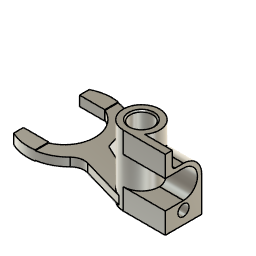
22 (Autodesk Fusion 360 design; units mm, degrees)
Autodesk Fusion 360 part; units mm, degrees
note: some values were not read from the file. Chosen so that the rebuilt part matches the saved one: where a step ends.
sketch "草图1" plane through (0, 0, 0) normal (0, 0, 1) x (1, 0, 0)
  line L0 (-13.1652, 20) -> (4.8348, 20)
  line L1 (-13.1652, -20) -> (4.8348, -20)
  line L2 (-40, 0) -> (55, 0) construction
  line L3 (-13.1652, 20) -> (-13.1652, 26.957)
  line L4 (-13.1652, -20) -> (-13.1652, -26.957)
  line L5 (-13.1652, -20) -> (4.8348, -20)
  line L6 (4.8348, -20) -> (4.8348, -29.6078)
  line L7 (4.8348, 20) -> (4.8348, 29.6078)
  arc A0 (-13.1652, -26.957) -> (-13.1652, 26.957) centre (0, 0) ccw
  arc A1 (4.8348, -20.1481) -> (4.8348, 20.1481) centre (-4, 0) ccw
  line L8 (13.7832, 26.6462) -> (71.9727, -3.4533)
  line L9 (62.4167, -27.4964) -> (31.174, -18.5377)
  arc A2 (31.174, -18.5377) -> (21.3132, -21.1127) centre (28.4176, -28.1503) ccw
  circle A3 centre (66, -15) radius 13
  circle A4 centre (66, -15) radius 8
  point P0 (66, -15)
  dimension "d5" = 60
  dimension "d6" = 44
  dimension "d7" = 4
  dimension "d8" = 20
  dimension "d9" = 40
  dimension "d10" = 18
  dimension "d11" = 18
  dimension "d13" = 15
  dimension "d14" = 10
  dimension "d16" = 70
  dimension "d17" = 26
  dimension "d18" = 16
  dimension "d19" = 16
  constraint coincident A0.centre origin
  constraint horizontal L0
  constraint parallel L0 L1
  constraint horizontal L2
  constraint collinear A1.centre L2.start L2.end
  constraint perpendicular L0 L3
  constraint perpendicular L1 L4
  constraint coincident L6.end A0
  constraint perpendicular L1 L6
  constraint coincident L7.end A0
  constraint perpendicular L0 L7
  constraint coincident L7 A1.end
  constraint coincident L6 A1.start
  constraint coincident A0 L8.start
  constraint coincident A0 A2.end
  constraint tangent L9 A2
  constraint tangent A0 L8
  constraint tangent A0 A2
  constraint coincident P0 A3.centre
  constraint coincident L8.end A3
  constraint tangent L8 A3
  constraint tangent L9 A3
  constraint coincident A3 L9.start
  constraint concentric A3 A4
  measures "d5" diameter of A0
  measures "d6" diameter of A1
  measures "d7" distance of A1.centre A0.centre
  measures "d8" distance of L0 L2
  measures "d9" vertical distance of L0.start L1.start
  measures "d10" distance of L0.start L0.end
  measures "d11" distance of L1.start L1.end
  measures "d13" vertical distance of A0.centre P0
  measures "d14" radius of A2
  measures "d16" horizontal distance of A1.centre P0
  measures "d17" diameter of A3
  measures "d18" angle of L2 L9
  measures "d19" diameter of A4
extrude "拉伸1" add sketch "草图1" along normal mid plane 7 contours L0 L3 L7 A0 | L1 L4 L5 L6 A0 makes body 1 at (-4.8402, -23.1181, 3.5) makes body 2 at (-4.8402, 23.1181, 3.5)
extrude "拉伸2" add sketch "草图1" along normal mid plane 6 contours L6 L7 A0 A1 | A0 L8 L9 A2 A3 bodies 1 2
extrude "拉伸3" add sketch "草图1" along normal blind 45.5 and the other way blind 4.5 contours A3 bodies 1
chamfer "倒角1" distance 1 angle 45 1 edges at (58.5414, -12.1071, 45.5) measured on face at (77.1299, -13.3248, 45.5) on bodies 1
ref_plane "工作平面1" through (66, 0, 0) normal (1, 0, 0) x (0, 1, 0)
sketch "草图2" plane through (66, 0, 0) normal (1, 0, 0) x (0, 1, 0)
  line L0 (-28, -4.5) -> (-2, -4.5)
  line L1 (-2, 45.5) -> (-28, 45.5)
  line L2 (-28, 45.5) -> (-23, 45.5)
  line L3 (-23, 45.5) -> (-23, 35.5)
  arc A0 (-23, 35.5) -> (-21, 33.5) centre (-21, 35.5) ccw
  line L4 (-21, 33.5) -> (-15, 33.5)
  arc A1 (-2, 20.5) -> (-15, 33.5) centre (-15, 20.5) ccw
  line L5 (-2, 20.5) -> (-2, -4.5)
  line L6 (-28, -4.5) -> (-28, 10.5)
  line L7 (-28, 10.5) -> (-15, 10.5)
  arc A2 (-15, 10.5) -> (-15, 30.5) centre (-15, 20.5) ccw
  line L8 (-15, 30.5) -> (-28, 30.5)
  line L9 (-28, 30.5) -> (-28, 45.5)
  circle A3 centre (-15, 4.5) radius 4
  point P0 (-15, 45.5)
  point P1 (-15, -4.5)
  dimension "d31" = 5
  dimension "d32" = 2
  dimension "d33" = 10
  dimension "d34" = 13
  dimension "d35" = 25
  dimension "d36" = 8
  dimension "d37" = 9
  constraint coincident L1.end L2.start
  constraint coincident L1 L2.end
  constraint perpendicular L2 L3
  constraint tangent L3 A0
  constraint perpendicular L3 L4
  constraint tangent L4 A1
  constraint coincident L0.end L5.end
  constraint coincident L0.start L6.start
  constraint perpendicular L0 L6
  constraint perpendicular L6 L7
  constraint tangent L7 A2
  constraint tangent A2 L8
  constraint perpendicular L6 L8
  constraint perpendicular L2 L9
  constraint tangent A0 L4
  constraint coincident A1.centre A2.centre
  constraint midpoint L1 P0
  constraint midpoint L0 P1
  constraint collinear A1.centre P0 P1
  constraint vertical L5
  constraint collinear P0 P1 A3.centre
  measures "d31" distance of L1.end L2.end
  measures "d32" radius of A0
  measures "d33" radius of A2
  measures "d34" radius of A1
  measures "d35" distance of A1.centre P1
  measures "d36" diameter of A3
  measures "d37" distance of P1 A3.centre
ref_plane "工作平面2" through (96, 0, 0) normal (1, 0, 0) x (0, 1, 0)
sketch "草图3" plane through (96, 0, 0) normal (1, 0, 0) x (0, 1, 0)
  line L0 (-28, -4.5) -> (-28, 10.5)
  line L1 (-28, 10.5) -> (-15, 10.5)
  arc A0 (-15, 10.5) -> (-15, 30.5) centre (-15, 20.5) ccw
  line L2 (-15, 30.5) -> (-28, 30.5)
  line L3 (-28, 45.5) -> (-23, 45.5)
  arc A1 (-23, 35.5) -> (-21, 33.5) centre (-21, 35.5) ccw
  line L4 (-21, 33.5) -> (-15, 33.5)
  arc A2 (-2, 20.5) -> (-15, 33.5) centre (-15, 20.5) ccw
  line L5 (-2, 20.5) -> (-2, -4.5)
  line L6 (-23, 45.5) -> (-23, 35.5)
  line L7 (-28, -4.5) -> (-2, -4.5)
  circle A3 centre (-15, 4.5) radius 4
  line L8 (-28, 30.5) -> (-28, 45.5)
extrude "拉伸4" add sketch "草图3" along normal up to near side of body 1 bodies 1
extrude "拉伸5" cut sketch "草图3" along normal up to surface contours A3 end surface at (73.9602, -15.7965, 11.8333) on bodies 1 bodies 1
sketch "草图4" plane through (0, 0, 3) normal (0, 0, 1) x (-1, 0, 0)
  line L0 (-66, 2) -> (-69.1632, 2)
  line L1 (-69.1632, 2) -> (-13.7832, -26.6462)
  arc A0 (-13.7832, -26.6462) -> (-4.8348, -29.6078) centre (0, 0) ccw
  line L2 (-4.8348, -29.6078) -> (-4.8348, -20.1481)
  arc A1 (-4.8348, 20.1481) -> (-4.8348, -20.1481) centre (4, 0) ccw
  line L3 (-4.8348, 20.1481) -> (-4.8348, 29.6078)
  arc A2 (-4.8348, 29.6078) -> (-21.3132, 21.1127) centre (0, 0) ccw
  arc A3 (-31.174, 18.5377) -> (-21.3132, 21.1127) centre (-28.4176, 28.1503) ccw
  line L4 (-31.174, 18.5377) -> (-62.4167, 27.4964)
  arc A4 (-66, 2) -> (-62.4167, 27.4964) centre (-66, 15) ccw
  line L5 (-66, 15) -> (-28.1042, -2.6711)
  line L6 (0, 0) -> (-100, 0) construction
  dimension "d43" = 25
  constraint coincident A4.centre L5.start
  constraint coincident A0.centre A2.centre
  constraint parallel L0 L6
  measures "d43" angle of L5 L6
sketch "草图5" plane through (0, 0, 45.5) normal (0, 0, 1) x (-1, 0, 0)
  arc A0 (-76.247, 23) -> (-66, 28) centre (-66, 15) ccw
  line L0 (-66, 28) -> (-96, 28)
  line L1 (-96, 28) -> (-96, 23)
  line L2 (-96, 23) -> (-76.247, 23)
  circle A1 centre (-66, 15) radius 9
  point P0 (-66, 15)
  constraint coincident P0 A0.centre
ref_plane "工作平面3" through (66, -15, 45.5) normal (0.422618, 0.906308, 0) x (-0.906308, 0.422618, 0)
sketch "草图6" plane through (6.0427, 12.9586, 0) normal (0.422618, 0.906308, 0) x (-0.906308, 0.422618, 0)
  line L0 (-26.1556, 3) -> (-56.1556, 37)
  line L1 (-56.1556, 37) -> (-56.1556, 3)
  line L2 (-56.1556, 3) -> (-26.1556, 3)
  point P0 (-66.1556, 45.5)
  point P1 (-66.1556, 3)
  point P2 (-24.3421, 3)
  dimension "d44" = 40
  dimension "d45" = 34
  dimension "d46" = 30
  constraint horizontal L2
  constraint collinear P1 P2 L0.start
  constraint vertical L1
  measures "d44" horizontal distance of P0 L0.start
  measures "d45" distance of L0.end L1.end
  measures "d46" distance of L0.start L1.end
extrude "拉伸6" add sketch "草图6" along normal mid plane 6 bodies 1
